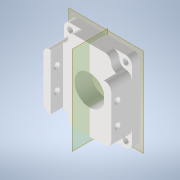
# Autodesk Inventor part: ESP32ParasiteMicroscope_sample_v1
Saved by Autodesk Inventor 2022 (Build 260153000, 153)
## iProperties
Created: 2022-03-06
Part Number: ESP32ParasiteMicroscope_sample_v1
Material: Generic
Document SubType Name: Modeling
Designer: Prakash Lab
Density: 1 g/cm^3
Appearance: Default
Author: Prakash Lab
Autodesk Inventor part; units mm, degrees
ref_plane "YZ Plane" through (0, 0, 0) normal (1, 0, 0) x (0, 1, 0)
ref_plane "XZ Plane" through (0, 0, 0) normal (0, 1, 0) x (-1, 0, 0)
ref_plane "Work Plane1" through (0, 0, 0) normal (0, 0, 1) x (1, 0, 0)
sketch "Sketch1" plane through (0, 0, 0) normal (0, 0, 1) x (1, 0, 0)
  circle A0 centre (-13.4362, 16.4874) radius 1.45 projected
  circle A1 centre (13.4362, 16.4874) radius 1.45 projected
  circle A2 centre (13.4362, -16.4874) radius 1.45 projected
  circle A3 centre (-13.4362, -16.4874) radius 1.45 projected
  line L0 (-16.4362, 16.4874) -> (-16.4362, -16.4874) projected
  arc A4 (-16.4362, -16.4874) -> (-13.4362, -19.4874) centre (-13.4362, -16.4874) ccw projected
  line L1 (-13.4362, -19.4874) -> (13.4362, -19.4874) projected
  arc A5 (13.4362, -19.4874) -> (16.4362, -16.4874) centre (13.4362, -16.4874) ccw projected
  line L2 (16.4362, -16.4874) -> (16.4362, 16.4874) projected
  arc A6 (16.4362, 16.4874) -> (13.4362, 19.4874) centre (13.4362, 16.4874) ccw projected
  line L3 (13.4362, 19.4874) -> (-13.4362, 19.4874) projected
  arc A7 (-13.4362, 19.4874) -> (-16.4362, 16.4874) centre (-13.4362, 16.4874) ccw projected
  arc A8 (-1.5588, 6.4) -> (-6.322, -1.85) centre (-1.5588, 0.9) ccw projected
  line L4 (1.5588, 6.4) -> (-1.5588, 6.4) projected
  arc A9 (6.322, -1.85) -> (1.5588, 6.4) centre (1.5588, 0.9) ccw projected
  line L5 (4.7631, -4.55) -> (6.322, -1.85) projected
  arc A10 (-4.7631, -4.55) -> (4.7631, -4.55) centre (0, -1.8) ccw projected
  line L6 (-6.322, -1.85) -> (-4.7631, -4.55) projected
  circle A11 centre (0, 0) radius 7.3
  constraints: 1 centre point, 1 coincident
ref_plane "Work Plane2" through (-15.9247, -43.8235, 15.65) normal (0, 0, -1) x (0, 1, 0)
extrude "Extrusion1" add sketch "Sketch1" along normal blind 8
ref_plane "Work Plane3" through (0, -16.4874, 0) normal (-1, 0, 0) x (0, 0, 1)
sketch "Sketch2" plane through (-13.4362, -19.4874, 8) normal (0, 0, 1) x (1, 0, 0)
  circle A0 centre (0, 35.9749) radius 1.45 projected
  circle A1 centre (26.8724, 35.9749) radius 1.45 projected
  circle A2 centre (26.8724, 3) radius 1.45 projected
  circle A3 centre (0, 3) radius 1.45 projected
  point P0 (13.4362, 19.4874)
hole "Hole1" at (-13.4362, 16.4874, 8) at (13.4362, 16.4874, 8) at (13.4362, -16.4874, 8) at (-13.4362, -16.4874, 8) direction (0, 0, -1) diameter 2.9 depth 15 tip angle 118 counterbore diameter 6 counterbore depth 4
fillet "Fillet1" radius 3.175 8 edges at (16.4362, -16.4874, 6) (13.4362, -19.4874, 6) (-13.4362, -19.4874, 6) (-16.4362, -16.4874, 6) (-13.4362, 19.4874, 6) (-16.4362, 16.4874, 6) (16.4362, 16.4874, 6) (13.4362, 19.4874, 6)
sketch "Sketch3" plane through (-7.2637, 19.4874, 8) normal (0, 0, 1) x (1, 0, 0)
  line L0 (-5.4363, 18.0594) -> (-5.4363, -57.4406) projected
  line L1 (19.9637, -57.4406) -> (19.9637, 18.0594) projected
  arc A0 (-3.1737, -35.8899) -> (-6.0875, -32.9761) centre (-6.1725, -35.9749) ccw projected
  arc A1 (-9.1725, -29.8024) -> (-6.0875, -32.9761) centre (-5.9975, -29.8024) ccw projected
  line L2 (-9.1725, -29.8024) -> (-9.1725, -35.9749) projected
  arc A2 (-9.1725, -35.9749) -> (-6.1725, -38.9749) centre (-6.1725, -35.9749) ccw projected
  line L3 (-6.1725, -38.9749) -> (0, -38.9749) projected
  arc A3 (-3.1737, -35.8899) -> (0, -38.9749) centre (0, -35.7999) ccw projected
  circle A4 centre (-6.1725, -35.9749) radius 1.45 projected
  arc A5 (-6.0875, -5.9988) -> (-3.1737, -3.085) centre (-6.1725, -3) ccw projected
  arc A6 (0, 0) -> (-3.1737, -3.085) centre (0, -3.175) ccw projected
  line L4 (0, 0) -> (-6.1725, 0) projected
  arc A7 (-6.1725, 0) -> (-9.1725, -3) centre (-6.1725, -3) ccw projected
  line L5 (-9.1725, -3) -> (-9.1725, -9.1725) projected
  arc A8 (-6.0875, -5.9988) -> (-9.1725, -9.1725) centre (-5.9975, -9.1725) ccw projected
  circle A9 centre (-6.1725, -3) radius 1.45 projected
  arc A10 (23.6998, -3) -> (20.6998, 0) centre (20.6998, -3) ccw projected
  line L6 (20.6998, 0) -> (14.5273, 0) projected
  arc A11 (17.701, -3.085) -> (14.5273, 0) centre (14.5273, -3.175) ccw projected
  arc A12 (17.701, -3.085) -> (20.6148, -5.9988) centre (20.6998, -3) ccw projected
  arc A13 (23.6998, -9.1725) -> (20.6148, -5.9988) centre (20.5248, -9.1725) ccw projected
  line L7 (23.6998, -9.1725) -> (23.6998, -3) projected
  circle A14 centre (20.6998, -3) radius 1.45 projected
  arc A15 (20.6148, -32.9761) -> (17.701, -35.8899) centre (20.6998, -35.9749) ccw projected
  arc A16 (14.5273, -38.9749) -> (17.701, -35.8899) centre (14.5273, -35.7999) ccw projected
  line L8 (14.5273, -38.9749) -> (20.6998, -38.9749) projected
  arc A17 (20.6998, -38.9749) -> (23.6998, -35.9749) centre (20.6998, -35.9749) ccw projected
  line L9 (23.6998, -35.9749) -> (23.6998, -29.8024) projected
  arc A18 (20.6148, -32.9761) -> (23.6998, -29.8024) centre (20.5248, -29.8024) ccw projected
  circle A19 centre (20.6998, -35.9749) radius 1.45 projected
  line L10 (-5.6363, -5.9517) -> (-5.6363, -33.0232)
  arc A20 (-3.1737, -35.8899) -> (-6.0875, -32.9761) centre (-6.1725, -35.9749) ccw projected
  line L11 (20.1637, -33.0232) -> (20.1637, -5.9517)
  arc A21 (17.701, -3.085) -> (20.6148, -5.9988) centre (20.6998, -3) ccw projected
  arc A22 (20.6148, -32.9761) -> (17.701, -35.8899) centre (20.6998, -35.9749) ccw projected
  arc A23 (-6.0875, -5.9988) -> (-3.1737, -3.085) centre (-6.1725, -3) ccw projected
  line L12 (-9.1725, -9.1725) -> (-9.1725, -29.8024)
  line L13 (23.6998, -29.8024) -> (23.6998, -9.1725) projected
  line L14 (23.6998, -9.1725) -> (23.6998, -29.8024)
  point P0 (7.2637, -19.4874)
  point P1 (-5.6363, -33.0232)
  point P2 (-5.6363, -5.9517)
  point P3 (20.1637, -5.9517)
  dimension "d10" = 0.2
  dimension "d11" = 0.2
  constraints: 8 end point, 4 point on circle, 4 vertical, 2 parallel
  measures "d10" distance between parallel lines of L1 L11
  measures "d11" distance between parallel lines of L10 L0
extrude "Extrusion2" add sketch "Sketch3" along normal blind 6 contours A8 A5 L10 A0 A1 L12 | A18 A15 L11 A12 A13 L13
sketch "Sketch4" plane through (-16.4362, -16.4874, 0) normal (-1, 0, 0) x (0, 0, 1)
  line L0 (0, 32.9749) -> (4, 32.9749) projected
  line L1 (0, 32.9749) -> (0, 0) projected
  line L2 (0, 0) -> (4, 0) projected
  circle A0 centre (11, 21.8024) radius 1.45
  circle A1 centre (11, 11.1725) radius 1.45
  line L3 (4, 32.9749) -> (4, 26.8024) projected
  line L4 (4, 6.1725) -> (4, 0) projected
  line L5 (14, 6.1725) -> (4, 6.1725) projected
  line L6 (4, 26.8024) -> (14, 26.8024) projected
  line L7 (14, 26.8024) -> (14, 6.1725) projected
  line L8 (8, 32.8899) -> (8, 30.0232) projected
  point P0 (0, 16.4874)
  dimension "d14" = 2.9
  dimension "d15" = 2.9
  dimension "d22" = 3
  dimension "d23" = 0
  constraints: 2 centre point
  measures "d14" diameter of A0
  measures "d15" diameter of A1
  measures "d22" distance from line of L8 A0.centre
  measures "d23" horizontal distance of A1.centre A0.centre
extrude "Extrusion3" cut sketch "Sketch4" against normal through all contours A0 | A1
body "Solid1"
